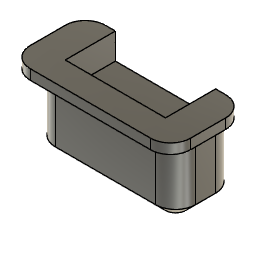
Button_V1 (Autodesk Fusion 360 design; units mm, degrees)
Autodesk Fusion 360 part; units mm, degrees
sketch "Sketch1" plane through (0, 0, 0) normal (0, 0, 1) x (1, 0, 0)
  line L0 (1, 0) -> (6, 0)
  line L1 (7, 1) -> (7, 2)
  line L2 (6, 3) -> (1, 3)
  line L3 (0, 2) -> (0, 1)
  arc A0 (1, 3) -> (0, 2) centre (1, 2) ccw
  arc A1 (0, 1) -> (1, 0) centre (1, 1) ccw
  arc A2 (7, 2) -> (6, 3) centre (6, 2) ccw
  arc A3 (6, 0) -> (7, 1) centre (6, 1) ccw
  point P0 (7, 3)
  point P1 (0, 3)
  dimension "d1" = 7
  dimension "d2" = 3
  dimension "d3" = 1
  constraint horizontal L0
  constraint vertical L1
  constraint horizontal L2
  constraint vertical L3
  constraint coincident P1 L2
  constraint coincident P1 L3
  constraint tangent L2 A0
  constraint tangent L3 A0
  constraint coincident origin L0
  constraint coincident origin L3
  constraint tangent L0 A1
  constraint tangent L3 A1
  constraint equal A0 A1
  constraint coincident P0 L1
  constraint coincident P0 L2
  constraint tangent L1 A2
  constraint tangent L2 A2
  constraint equal A0 A2
  constraint tangent L0 A3
  constraint tangent L1 A3
  constraint equal A0 A3
  measures "d1" distance of P0 P1
  measures "d2" distance of origin P1
  measures "d3" radius of A0
extrude "Extrude1" add sketch "Sketch1" along normal blind 3.5
sketch "Sketch2" plane through (0, 0, 3.5) normal (0, 0, 1) x (-1, 0, 0)
  arc A0 (-6, 0) -> (-7, -1) centre (-6, -1) ccw
  line L0 (-7, -1) -> (-7, -2)
  arc A1 (-7, -2) -> (-6, -3) centre (-6, -2) ccw
  line L1 (-6, -3) -> (-1, -3)
  arc A2 (-1, -3) -> (0, -2) centre (-1, -2) ccw
  line L2 (0, -2) -> (0, -1)
  arc A3 (0, -1) -> (-1, 0) centre (-1, -1) ccw
  line L3 (-1, 0) -> (-6, 0)
  line L4 (-0.5, -3) -> (-6.5, -3)
  line L5 (-7.5, -2) -> (-7.5, -0.25)
  line L6 (-6.5, 0.75) -> (-0.5, 0.75)
  line L7 (0.5, -0.25) -> (0.5, -2)
  arc A4 (0.5, -0.25) -> (-0.5, 0.75) centre (-0.5, -0.25) ccw
  arc A5 (-6.5, 0.75) -> (-7.5, -0.25) centre (-6.5, -0.25) ccw
  arc A6 (-0.5, -3) -> (0.5, -2) centre (-0.5, -2) ccw
  arc A7 (-7.5, -2) -> (-6.5, -3) centre (-6.5, -2) ccw
  dimension "d6" = 0.5
  dimension "d7" = 0.5
  dimension "d8" = 0.75
  dimension "d11" = 1
  constraint horizontal L4
  constraint vertical L5
  constraint horizontal L6
  constraint vertical L7
  constraint tangent L6 A4
  constraint tangent L7 A4
  constraint tangent L5 A5
  constraint tangent L6 A5
  constraint equal A4 A5
  constraint tangent L4 A6
  constraint tangent L7 A6
  constraint equal A4 A6
  constraint tangent L4 A7
  constraint tangent L5 A7
  constraint equal A4 A7
  measures "d6" distance of L2 L7
  measures "d7" distance of L0 L5
  measures "d8" distance of L3 L6
  measures "d11" radius of A4
extrude "Extrude2" add sketch "Sketch2" along normal blind 0.5
chamfer "Chamfer1" distance 0.5 angle 45 8 edges at (0, 1.5, 0) (0.2929, 0.2929, 0) (3.5, 0, 0) (6.7071, 0.2929, 0) (7, 1.5, 0) (6.7071, 2.7071, 0) (3.5, 3, 0) (0.2929, 2.7071, 0)
sketch "Sketch3" plane through (0, 3, 0) normal (0, 1, 0) x (-1, 0, 0)
  line L0 (-6, 0.5) -> (-1, 0.5)
  line L1 (-1, 0.5) -> (-1, 3.5)
  line L2 (-0.5, 4) -> (-6.5, 4)
  line L3 (-6, 3.5) -> (-6, 0.5)
  line L4 (-5.9973, 4) -> (-0.9973, 4)
  line L5 (-0.9973, 4) -> (-0.9973, 2.7)
  line L6 (-0.9973, 2.7) -> (-5.9973, 2.7)
  line L7 (-5.9973, 2.7) -> (-5.9973, 4)
  line L8 (-1, 3.5) -> (-0.5, 3.5)
  line L9 (-0.5, 3.5) -> (-0.5, 4)
  line L10 (-6.5, 4) -> (-6.5, 3.5)
  line L11 (-6.5, 3.5) -> (-6, 3.5)
  dimension "d13" = 5
  dimension "d20" = 1.3
  constraint horizontal L4
  constraint vertical L5
  constraint horizontal L6
  constraint vertical L7
  constraint coincident L2 L4.start
  measures "d13" distance of L5.end L6.end
  measures "d20" distance of L4.end L5.end
extrude "Extrude3" cut sketch "Sketch3" against normal blind 2.5 contours L1 L2 L3 L4 L5 L6 L7
